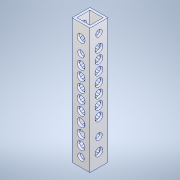
# Autodesk Inventor part: ハンド9x9_4
Saved by Autodesk Inventor 2020.3 (Build 243373000, 373)
## iProperties
Created: 2020-05-31
Part Number: ハンド9x9_4
Material: アルミニウム 6061
Document SubType Name: Modeling
Designer: totot
Mass: 4.76254 g
Surface Area: 36.2695 cm^2
Volume: 1.7639 cm^3
Density: 2.7 g/cm^3
Appearance: アルミニウム - フラット
Author: totot
Autodesk Inventor part; units mm, degrees
ref_plane "YZ Plane" through (0, 0, 0) normal (1, 0, 0) x (0, 1, 0)
ref_plane "XZ Plane" through (0, 0, 0) normal (0, 1, 0) x (-1, 0, 0)
ref_plane "XY Plane" through (0, 0, 0) normal (0, 0, 1) x (1, 0, 0)
sketch "スケッチ1" plane through (0, 0, 0) normal (0, 1, 0) x (-1, 0, 0)
  line L0 (0, 0) -> (-9, 0)
  line L1 (-9, 0) -> (-9, -9)
  line L2 (-9, -9) -> (0, -9)
  line L3 (0, -9) -> (0, 0)
  line L4 (-1.2, -1.2) -> (-7.8, -1.2)
  line L5 (-7.8, -1.2) -> (-7.8, -7.8)
  line L6 (-7.8, -7.8) -> (-1.2, -7.8)
  line L7 (-1.2, -7.8) -> (-1.2, -1.2)
  dimension "d0" = 9
  dimension "d1" = 9
  dimension "d2" = 1.2
  dimension "d3" = 1.2
  dimension "d4" = 1.2
  dimension "d5" = 1.2
  constraints: 16 end point, 4 parallel, 2 horizontal, 2 perpendicular
  measures "d0" distance of L0.start L0.end
  measures "d1" distance of L2.end L0.start
  measures "d2" distance between parallel lines of L0 L4
  measures "d3" distance between parallel lines of L7 L3
  measures "d4" distance between parallel lines of L6 L2
  measures "d5" distance between parallel lines of L1 L5
extrude "押し出し1" add sketch "スケッチ1" along normal blind 63
sketch "スケッチ2" plane through (9, 0, 0) normal (1, 0, 0) x (0, 0, -1)
  line L0 (0, 63) -> (9, 63) projected
  line L1 (9, 0) -> (9, 63) projected
  line L2 (0, 0) -> (9, 0) projected
  point P0 (4.5, 58.5)
  point P1 (4.5, 13.5)
  dimension "d8" = 4.5
  dimension "d9" = 4.5
  dimension "d10" = 4.5
  dimension "d11" = 13.5
  measures "d8" distance from line of point (4.5, 58.5) L0
  measures "d9" distance from line of point (4.5, 58.5) L1
  measures "d10" distance from line of L1 point (4.5, 13.5)
  measures "d11" distance from line of L2 point (4.5, 13.5)
hole "穴1" at (9, 58.5, -4.5) at (9, 13.5, -4.5) direction (-1, 0, 0) diameter 3.3 end through all
sketch "スケッチ3" plane through (0, 0, 0) normal (0, 0, 1) x (1, 0, 0)
  line L0 (0, 0) -> (0, 63) projected
  line L1 (0, 0) -> (9, 0) projected
  line L2 (0, 63) -> (9, 63) projected
  point P0 (4.5, 49.5)
  point P1 (4.5, 4.5)
  dimension "d19" = 4.5
  dimension "d20" = 4.5
  dimension "d21" = 13.5
  dimension "d22" = 4.5
  measures "d19" distance from line of L0 point (4.5, 4.5)
  measures "d20" distance from line of point (4.5, 4.5) L1
  measures "d21" distance from line of point (4.5, 49.5) L2
  measures "d22" distance from line of L0 point (4.5, 49.5)
hole "穴2" at (4.5, 49.5, 0) at (4.5, 4.5, 0) direction (0, 0, -1) diameter 3.3 end through all
sketch "スケッチ4" plane through (9, 0, 0) normal (1, 0, 0) x (0, 0, -1)
  line L0 (0, 0) -> (9, 0) projected
  line L1 (9, 0) -> (9, 63) projected
  point P0 (4.5, 22)
  dimension "d30" = 22
  dimension "d31" = 4.5
  measures "d30" distance from line of point (4.5, 22) L0
  measures "d31" distance from line of point (4.5, 22) L1
hole "穴3" at (9, 22, -4.5) direction (-1, 0, 0) diameter 4 end through all
sketch "スケッチ5" plane through (0, 0, 0) normal (0, 0, 1) x (1, 0, 0)
  line L0 (0, 63) -> (9, 63) projected
  line L1 (9, 0) -> (9, 63) projected
  circle A0 centre (4.5, 49.5) radius 1.65 projected
  point P0 (0, 0)
  point P1 (4.5, 56.25)
  point P2 (4.5, 44.5)
  point P3 (4.5, 39.5)
  point P4 (4.5, 34.5)
  point P5 (4.5, 29.5)
  point P6 (4.5, 24.5)
  point P7 (4.5, 19.5)
  point P8 (4.5, 14.5)
  point P9 (4.5, 9.5)
  dimension "d39" = 6.75
  dimension "d40" = 4.5
  dimension "d41" = 4.5
  dimension "d42" = 5
  dimension "d45" = 5
  constraints: 1 vertical, 7 other
  measures "d39" distance from line of point (4.5, 56.25) L0
  measures "d40" distance from line of point (4.5, 56.25) L1
  measures "d41" distance from line of L1 point (4.5, 44.5)
  measures "d42" distance of point (4.5, 44.5) A0.centre
  measures "d45" distance of point (4.5, 44.5) point (4.5, 39.5)
hole "穴4" at (4.5, 56.25, 0) at (4.5, 44.5, 0) at (4.5, 39.5, 0) at (4.5, 34.5, 0) at (4.5, 29.5, 0) at (4.5, 24.5, 0) at (4.5, 19.5, 0) at (4.5, 14.5, 0) at (4.5, 9.5, 0) direction (0, 0, -1) diameter 4 end through all
sketch "スケッチ7" plane through (9, 0, 0) normal (1, 0, 0) x (0, 0, -1)
  line L0 (0, 0) -> (0, 63) projected
  line L1 (0, 0) -> (9, 0) projected
  circle A0 centre (4.5, 22) radius 2 projected
  point P0 (4.5, 6.75)
  point P1 (4.5, 27)
  point P2 (4.5, 32)
  point P3 (4.5, 37)
  point P4 (4.5, 42)
  point P5 (4.5, 47)
  point P6 (4.5, 52)
  dimension "d57" = 4.5
  dimension "d58" = 4.5
  dimension "d59" = 6.75
  dimension "d60" = 5
  dimension "d63" = 5
  constraints: 1 vertical, 5 other
  measures "d57" distance from line of L0 point (4.5, 27)
  measures "d58" distance from line of L0 point (4.5, 6.75)
  measures "d59" distance from line of L1 point (4.5, 6.75)
  measures "d60" distance of A0.centre point (4.5, 27)
  measures "d63" distance of point (4.5, 27) point (4.5, 32)
hole "穴5" at (9, 6.75, -4.5) at (9, 27, -4.5) at (9, 32, -4.5) at (9, 37, -4.5) at (9, 42, -4.5) at (9, 47, -4.5) at (9, 52, -4.5) direction (-1, 0, 0) diameter 4 end through all
equation "\"d4\" = d3"
equation "\"d5\" = d4"
equation "\"d9\" = d8"
equation "\"d10\" = d9"
equation "\"d20\" = d19"
equation "\"d22\" = d19"
equation "\"d58\" = d57"
